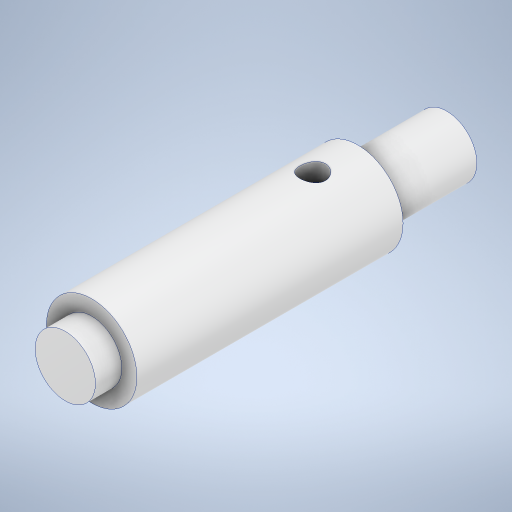
# Autodesk Inventor part: install-encoder-v1-Shaft-E-Shaft
Saved by Autodesk Inventor 2024.1 (Build 281209000, 209)
## iProperties
Created: 2024-02-12
Part Number: install-encoder-v1-Shaft-E-Shaft
Material: アルミニウム 6061
Document SubType Name: Modeling
Designer: haruy
Density: 2.7 g/cm^3
Appearance: アルミニウム - フラット
Author: haruy
Autodesk Inventor part; units mm, degrees
ref_plane "YZ Plane" through (0, 0, 0) normal (1, 0, 0) x (0, 1, 0)
ref_plane "XY Plane" through (0, 0, 0) normal (0, 0, 1) x (1, 0, 0)
sketch "スケッチ2" plane through (0, 0, 0) normal (1, 0, 0) x (0, 1, 0)
  line L0 (0, 0) -> (6, 0)
  line L1 (6, 0) -> (6, -50.65)
  line L2 (6, -50.65) -> (0, -50.65)
  line L3 (0, -50.65) -> (0, 0)
  line L4 (6, 0) -> (4, 0)
  line L5 (4, 0) -> (4, -3.5)
  line L6 (4, -3.5) -> (6, -3.5)
  line L7 (6, -3.5) -> (6, 0)
  line L8 (6, -50.65) -> (4, -50.65)
  line L9 (4, -50.65) -> (4, -38.85)
  line L10 (4, -38.85) -> (6, -38.85)
  line L11 (6, -38.85) -> (6, -50.65)
  dimension "d3" = 6
  dimension "d4" = 50.65
  dimension "d5" = 2
  dimension "d6" = 3.5
  dimension "d7" = 2
  dimension "d8" = 11.8
  constraints: 24 end point, 6 parallel, 3 horizontal, 3 perpendicular
  measures "d3" distance of L1.end L2.end
  measures "d4" distance of L0.end L1.end
  measures "d5" distance of L6.end L5.end
  measures "d6" distance of L5.end L4.end
  measures "d7" distance of L9.end L10.end
  measures "d8" distance of L8.end L9.end
revolve "回転1" add sketch "スケッチ2" angle 360 about axis through (0, 0, -50.65) along (0, 0, 1) contours L0 L5 L6 L1 L10 L9 L2 L3
ref_plane "作業平面1" through (0, 6, -21.175) normal (0, 1, 0) x (-1, 0, 0)
sketch "スケッチ3" plane through (0, 6, -21.175) normal (0, 1, 0) x (-1, 0, 0)
  line L0 (4, 21.175) -> (-4, 21.175) projected
  point P0 (0, 21.175)
  point P1 (0, -11.675)
  dimension "d10" = 32.85
  measures "d10" distance from line of L0 point (0, -11.675)
hole "穴1" at (0, 6, -32.85) direction (0, -1, 0) diameter 3.4 end through all
